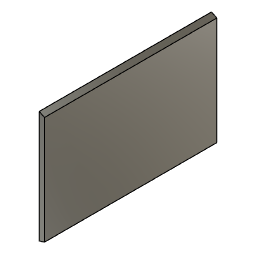
back2-top v3 (Autodesk Fusion 360 design; units mm, degrees)
Autodesk Fusion 360 part; units mm, degrees
note: some values were not read from the file. Set by a fixed rule: which sketch regions a step uses.
sketch "Esquisse1" plane through (0, 0, 0) normal (0, 1, 0) x (1, 0, 0)
  line L0 (0, -86.023) -> (0, 0)
  line L1 (4, -83.9629) -> (4, -1.2804)
  line L2 (0, 0) -> (4, -1.2804)
  line L3 (0, 0) -> (6.8882, 0) construction
  line L4 (0, -86.023) -> (4, -83.9629)
  dimension "d2" = 86.023
  dimension "d4" = 17.75
  dimension "d7" = 62.75
  constraint vertical L0
  constraint horizontal L3
  constraint coincident L0.end L2.start
  measures "d2" distance of L0.start L0.end
  measures "d4" angle of L2 L3
  measures "d7" angle of L0 L4
extrude "Extrusion1" add sketch "Esquisse1" along normal blind 132
